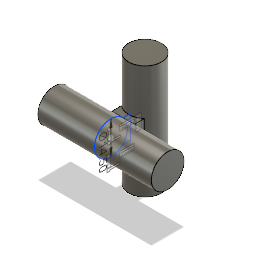
Joint_Assembly v7 (Autodesk Fusion 360 archive; units mm, degrees)
design "Dual_Elbow_Joint"
Autodesk Fusion 360 part; units mm, degrees
cylinder "CylinderPrimitive1" add diameter 14.5 height 50 placed x (1, 0, 0) y (0, 0, -1) z (0, 1, 0) at (0, 0, 0) makes body 1
sketch "Sketch6" plane through (0, 0, 0) normal (1, 0, 0) x (0, 0, -1)
  circle A0 centre (-15, 25) radius 7.25
  line L0 (-9.75, 30) -> (-6.3397, 30)
  line L1 (-6.3397, 30) -> (-6.3397, 19.8088)
  line L2 (-6.3397, 19.8088) -> (-9.939, 19.8088)
  dimension "d10" = 14.5
  constraint horizontal L0
  constraint vertical L1
  constraint horizontal L2
  constraint coincident A0 L0.start
  constraint coincident A0 L2.end
  measures "d10" diameter of A0
extrude "Extrude3" add sketch "Sketch6" along normal mid plane 10 contours A0 L0 L1 L2 bodies 1
extrude "Extrude2" add sketch "Sketch6" along normal mid plane 50 separate body contours A0 makes body 2
move_face "OffsetFaces1" offset 1 1 faces at (4.0114, 26.6029, 6.3397) on bodies 1
move_face "OffsetFaces2" offset 1 1 faces at (-4.5057, 26.6029, 6.3397) on bodies 1
